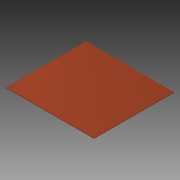
# Autodesk Inventor part: haetbed300
Saved by Autodesk Inventor 2013 (Build 170138000, 138)
## iProperties
Created: 2013-11-19
Part Number: haetbed300
Material: Generic
Document SubType Name: Modeling
Designer: Masta
Density: 1 g/cm^3
Author: Masta
Autodesk Inventor part; units mm, degrees
ref_plane "YZ Plane" through (0, 0, 0) normal (1, 0, 0) x (0, 1, 0)
ref_plane "XZ Plane" through (0, 0, 0) normal (0, 1, 0) x (-1, 0, 0)
ref_plane "XY Plane" through (0, 0, 0) normal (0, 0, 1) x (1, 0, 0)
sketch "Sketch1" plane through (0, 0, 0) normal (0, 0, 1) x (1, 0, 0)
  line L0 (-165, -150) -> (165, -150)
  line L1 (165, -150) -> (165, 150)
  line L2 (165, 150) -> (-165, 150)
  line L3 (-165, 150) -> (-165, -150)
  line L4 (-165, -150) -> (165, 150) construction
  line L5 (165, -150) -> (-165, 150) construction
  line L6 (-155, -140) -> (155, -140) construction
  line L7 (155, -140) -> (155, 140) construction
  line L8 (155, 140) -> (-155, 140) construction
  line L9 (-155, 140) -> (-155, -140) construction
  line L10 (-155, -140) -> (155, 140) construction
  line L11 (155, -140) -> (-155, 140) construction
  point P0 (0, 0)
  dimension "d0" = 330
  dimension "d1" = 300
  dimension "d4" = 310
  dimension "d5" = 280
  constraints: 24 end point, 4 coincident, 4 midpoint, 4 parallel, 2 horizontal, 2 perpendicular
  measures "d0" distance of L2.end L1.end
  measures "d1" distance of L1.end L0.end
  measures "d4" distance of L8.end L7.end
  measures "d5" distance of L7.end L6.end
extrude "Extrusion1" add sketch "Sketch1" along normal blind 1.5
hole "Hole1" at (-155, 140, 0) at (-155, -140, 0) at (155, -140, 0) at (155, 140, 0) direction (0, 0, 1) diameter 3 end through all
body "Solid1"
